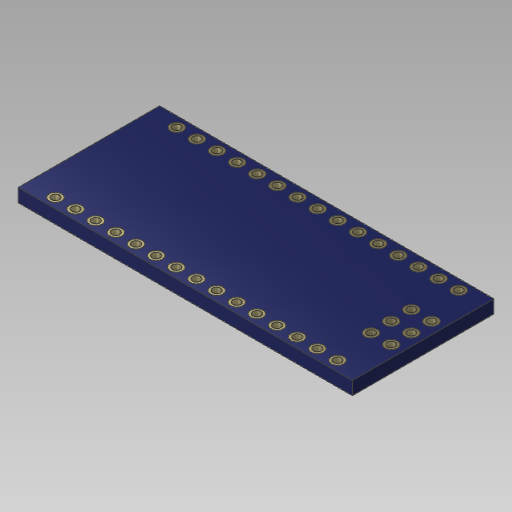
# Autodesk Inventor part: Arduino Nano
Saved by Autodesk Inventor 2020 (Build 240168000, 168)
## iProperties
Created: 2017-10-23
Part Number: Arduino Nano
Material: Generic
Document SubType Name: Modeling
Designer: Alex
Density: 1 g/cm^3
Appearance: Default
Author: Alex
Autodesk Inventor part; units mm, degrees
ref_plane "YZ Plane" through (0, 0, 0) normal (1, 0, 0) x (0, 1, 0)
ref_plane "XZ Plane" through (0, 0, 0) normal (0, 1, 0) x (-1, 0, 0)
ref_plane "XY Plane" through (0, 0, 0) normal (0, 0, 1) x (1, 0, 0)
sketch "Sketch1" plane through (0, 0, 0) normal (0, 1, 0) x (-1, 0, 0)
  line L0 (21.0693, -8.9154) -> (-21.0693, -8.9154)
  line L1 (-21.0693, -8.9154) -> (-21.0693, 8.9154)
  line L2 (-21.0693, 8.9154) -> (21.0693, 8.9154)
  line L3 (21.0693, 8.9154) -> (21.0693, -8.9154)
  line L4 (21.0693, -8.9154) -> (-21.0693, 8.9154) construction
  line L5 (-21.0693, -8.9154) -> (21.0693, 8.9154) construction
  point P0 (0, 0)
  dimension "d0" = 42.1386
  dimension "d1" = 17.8308
  constraints: 12 end point, 2 midpoint, 2 parallel, 1 horizontal, 1 perpendicular
  measures "d0" distance of L1.end L2.end
  measures "d1" distance of L0.end L1.end
extrude "Extrusion1" add sketch "Sketch1" along normal mid plane 1.651
sketch "Sketch2" plane through (0, 0.8255, 0) normal (0, 1, 0) x (1, 0, 0)
  circle A0 centre (-17.6403, 7.6454) radius 0.8001
  line L0 (-21.0693, 8.9154) -> (-21.0693, -8.9154) projected
  line L1 (21.0693, 8.9154) -> (-21.0693, 8.9154) projected
  line L2 (-21.0693, -8.9154) -> (21.0693, -8.9154) projected
  circle A1 centre (-15.1003, 7.6454) radius 0.8001
  circle A2 centre (-12.5603, 7.6454) radius 0.8001
  circle A3 centre (-10.0203, 7.6454) radius 0.8001
  circle A4 centre (-7.4803, 7.6454) radius 0.8001
  circle A5 centre (-4.9403, 7.6454) radius 0.8001
  circle A6 centre (-2.4003, 7.6454) radius 0.8001
  circle A7 centre (0.1397, 7.6454) radius 0.8001
  circle A8 centre (2.6797, 7.6454) radius 0.8001
  circle A9 centre (5.2197, 7.6454) radius 0.8001
  circle A10 centre (7.7597, 7.6454) radius 0.8001
  circle A11 centre (10.2997, 7.6454) radius 0.8001
  circle A12 centre (12.8397, 7.6454) radius 0.8001
  circle A13 centre (15.3797, 7.6454) radius 0.8001
  circle A14 centre (17.9197, 7.6454) radius 0.8001
  line L3 (0, 0) -> (-15.1003, 0) construction
  circle A15 centre (-17.6403, -7.6454) radius 0.8001
  circle A16 centre (-15.1003, -7.6454) radius 0.8001
  circle A17 centre (-12.5603, -7.6454) radius 0.8001
  circle A18 centre (-10.0203, -7.6454) radius 0.8001
  circle A19 centre (-7.4803, -7.6454) radius 0.8001
  circle A20 centre (-4.9403, -7.6454) radius 0.8001
  circle A21 centre (-2.4003, -7.6454) radius 0.8001
  circle A22 centre (0.1397, -7.6454) radius 0.8001
  circle A23 centre (2.6797, -7.6454) radius 0.8001
  circle A24 centre (5.2197, -7.6454) radius 0.8001
  circle A25 centre (7.7597, -7.6454) radius 0.8001
  circle A26 centre (10.2997, -7.6454) radius 0.8001
  circle A27 centre (12.8397, -7.6454) radius 0.8001
  circle A28 centre (15.3797, -7.6454) radius 0.8001
  circle A29 centre (17.9197, -7.6454) radius 0.8001
  circle A30 centre (19.5834, 0) radius 0.8001
  line L4 (21.0693, -8.9154) -> (21.0693, 8.9154) projected
  circle A31 centre (19.5834, -2.54) radius 0.8001
  circle A32 centre (17.0434, 0) radius 0.8001
  circle A33 centre (17.0434, -2.54) radius 0.8001
  circle A34 centre (17.0434, 2.54) radius 0.8001
  circle A35 centre (19.5834, 2.54) radius 0.8001
  dimension "d4" = 1.6002
  dimension "d5" = 3.429
  dimension "d6" = 1.27
  dimension "d7" = 17.8308
  dimension "d10" = 2.54
  dimension "d17" = 1.4859
  dimension "d21" = 2.54
  dimension "d24" = 2.54
  dimension "d29" = 2.54
  constraints: 36 centre point, 15 symmetric about line, 3 horizontal, 2 end point, 2 vertical, 1 equal radius, 1 horizontal alignment, 53 other
  measures "d4" diameter of A0
  measures "d5" distance from line of L0 A0.centre
  measures "d6" distance from line of L1 A0.centre
  measures "d7" distance between parallel lines of L2 L1
  measures "d10" distance of A0.centre A1.centre
  measures "d17" distance from line of L4 A30.centre
  measures "d21" distance of A30.centre A31.centre
  measures "d24" distance of A30.centre A32.centre
  measures "d29" distance of A32.centre A34.centre
extrude "Extrusion2" add sketch "Sketch2" along normal blind 0.0025 contours A0 | A1 | A2 | A3 | A4 | A5 | A6 | A7 | A8 | A9 | A10 | A11 | A12 | A13 | A14 | A15 | A16 | A17 | A18 | A19 | A20 | A21 | A22 | A23 | A24 | A25 | A26 | A27 | A28 | A29 | A30 | A31 | A32 | A33 | A34 | A35
mirror "Mirror1" about plane through (0, 0, 0) normal (0, 1, 0) of "Extrusion2"
sketch "Sketch4" plane through (-17.6403, 0.828, -7.6454) normal (0, 1, 0) x (1, 0, 0)
  circle A0 centre (34.6837, -5.1054) radius 0.8001 projected
  circle A1 centre (34.6837, -7.6454) radius 0.8001 projected
  circle A2 centre (37.2237, -7.6454) radius 0.8001 projected
  circle A3 centre (33.02, -15.2908) radius 0.8001 projected
  circle A4 centre (27.94, -15.2908) radius 0.8001 projected
  circle A5 centre (22.86, -15.2908) radius 0.8001 projected
  circle A6 centre (0, -15.2908) radius 0.8001 projected
  circle A7 centre (2.54, -15.2908) radius 0.8001 projected
  circle A8 centre (10.16, -15.2908) radius 0.8001 projected
  circle A9 centre (15.24, -15.2908) radius 0.8001 projected
  circle A10 centre (35.56, 0) radius 0.8001 projected
  circle A11 centre (30.48, 0) radius 0.8001 projected
  circle A12 centre (25.4, 0) radius 0.8001 projected
  circle A13 centre (20.32, 0) radius 0.8001 projected
  circle A14 centre (15.24, 0) radius 0.8001 projected
  circle A15 centre (10.16, 0) radius 0.8001 projected
  circle A16 centre (5.08, 0) radius 0.8001 projected
  circle A17 centre (0, 0) radius 0.8001 projected
  circle A18 centre (2.54, 0) radius 0.8001 projected
  circle A19 centre (7.62, 0) radius 0.8001 projected
  circle A20 centre (12.7, 0) radius 0.8001 projected
  circle A21 centre (17.78, 0) radius 0.8001 projected
  circle A22 centre (22.86, 0) radius 0.8001 projected
  circle A23 centre (27.94, 0) radius 0.8001 projected
  circle A24 centre (33.02, 0) radius 0.8001 projected
  circle A25 centre (17.78, -15.2908) radius 0.8001 projected
  circle A26 centre (12.7, -15.2908) radius 0.8001 projected
  circle A27 centre (7.62, -15.2908) radius 0.8001 projected
  circle A28 centre (5.08, -15.2908) radius 0.8001 projected
  circle A29 centre (20.32, -15.2908) radius 0.8001 projected
  circle A30 centre (25.4, -15.2908) radius 0.8001 projected
  circle A31 centre (30.48, -15.2908) radius 0.8001 projected
  circle A32 centre (35.56, -15.2908) radius 0.8001 projected
  circle A33 centre (37.2237, -10.1854) radius 0.8001 projected
  circle A34 centre (34.6837, -10.1854) radius 0.8001 projected
  circle A35 centre (37.2237, -5.1054) radius 0.8001 projected
  line L0 (38.7096, 1.27) -> (-3.429, 1.27) projected
  line L1 (-3.429, 1.27) -> (-3.429, -16.5608) projected
  line L2 (-3.429, -16.5608) -> (38.7096, -16.5608) projected
  line L3 (38.7096, -16.5608) -> (38.7096, 1.27) projected
  point P0 (17.6403, -7.6454)
hole "Hole1" at (0.1397, 0.828, 7.6454) at (2.6797, 0.828, 7.6454) at (-7.4803, 0.828, -7.6454) at (-2.4003, 0.828, -7.6454) at (-4.9403, 0.828, -7.6454) at (0.1397, 0.828, -7.6454) at (5.2197, 0.828, 7.6454) at (2.6797, 0.828, -7.6454) at (7.7597, 0.828, 7.6454) at (5.2197, 0.828, -7.6454) at (10.2997, 0.828, 7.6454) at (15.3797, 0.828, 7.6454) at (17.0434, 0.828, -2.54) at (-2.4003, 0.828, 7.6454) at (17.0434, 0.828, 0) at (19.5834, 0.828, 0) at (7.7597, 0.828, -7.6454) at (12.8397, 0.828, -7.6454) at (17.9197, 0.828, -7.6454) at (-17.6403, 0.828, 7.6454) at (-15.1003, 0.828, 7.6454) at (-10.0203, 0.828, 7.6454) at (-12.5603, 0.828, 7.6454) at (-10.0203, 0.828, -7.6454) at (-12.5603, 0.828, -7.6454) at (-15.1003, 0.828, -7.6454) at (-17.6403, 0.828, -7.6454) at (-7.4803, 0.828, 7.6454) at (-4.9403, 0.828, 7.6454) at (10.2997, 0.828, -7.6454) at (12.8397, 0.828, 7.6454) at (15.3797, 0.828, -7.6454) at (17.9197, 0.828, 7.6454) at (19.5834, 0.828, 2.54) at (19.5834, 0.828, -2.54) at (17.0434, 0.828, 2.54) direction (0, -1, 0) diameter 1.016 end through all
sketch "Sketch5" plane through (0, -0.8255, 0) normal (0, -1, 0) x (1, 0, 0)
  line L0 (-1.6129, 0) -> (-6.2611, 4.6482)
  line L1 (-6.2611, 4.6482) -> (-10.9093, 0)
  line L2 (-10.9093, 0) -> (-6.2611, -4.6482)
  line L3 (-6.2611, -4.6482) -> (-1.6129, 0)
  line L4 (-21.0693, 8.9154) -> (-21.0693, -8.9154) projected
  point P0 (0, 0)
  dimension "d45" = 9.2964
  dimension "d46" = 10.16
  constraints: 8 end point, 2 horizontal alignment, 2 parallel, 1 perpendicular, 1 vertical alignment
  measures "d45" distance of L1.end L0.start
  measures "d46" distance from line of L4 L1.end
extrude "Extrusion3" add sketch "Sketch5" along normal blind 1.143
sketch "Sketch6" plane through (-6.2611, -1.9685, -4.6482) normal (-0.7071, 0, -0.7071) x (-0.7071, 0, 0.7071)
  line L0 (0.508, 0.381) -> (0.889, 0.381)
  line L1 (0.889, 0.381) -> (0.889, 0.254)
  line L2 (0.889, 0.254) -> (0.508, 0.254)
  line L3 (0.508, 0.254) -> (0.508, 0.381)
  line L4 (6.5735, 0) -> (0, 0) projected
  line L5 (0, 1.143) -> (0, 0) projected
  line L6 (1.2475, 0.381) -> (1.6285, 0.381)
  line L7 (1.6285, 0.381) -> (1.6285, 0.254)
  line L8 (1.6285, 0.254) -> (1.2475, 0.254)
  line L9 (1.2475, 0.254) -> (1.2475, 0.381)
  line L10 (1.987, 0.381) -> (2.368, 0.381)
  line L11 (2.368, 0.381) -> (2.368, 0.254)
  line L12 (2.368, 0.254) -> (1.987, 0.254)
  line L13 (1.987, 0.254) -> (1.987, 0.381)
  line L14 (2.7265, 0.381) -> (3.1075, 0.381)
  line L15 (3.1075, 0.381) -> (3.1075, 0.254)
  line L16 (3.1075, 0.254) -> (2.7265, 0.254)
  line L17 (2.7265, 0.254) -> (2.7265, 0.381)
  line L18 (3.466, 0.381) -> (3.847, 0.381)
  line L19 (3.847, 0.381) -> (3.847, 0.254)
  line L20 (3.847, 0.254) -> (3.466, 0.254)
  line L21 (3.466, 0.254) -> (3.466, 0.381)
  line L22 (4.2055, 0.381) -> (4.5865, 0.381)
  line L23 (4.5865, 0.381) -> (4.5865, 0.254)
  line L24 (4.5865, 0.254) -> (4.2055, 0.254)
  line L25 (4.2055, 0.254) -> (4.2055, 0.381)
  line L26 (4.945, 0.381) -> (5.326, 0.381)
  line L27 (5.326, 0.381) -> (5.326, 0.254)
  line L28 (5.326, 0.254) -> (4.945, 0.254)
  line L29 (4.945, 0.254) -> (4.945, 0.381)
  line L30 (5.6845, 0.381) -> (6.0655, 0.381)
  line L31 (6.0655, 0.381) -> (6.0655, 0.254)
  line L32 (6.0655, 0.254) -> (5.6845, 0.254)
  line L33 (5.6845, 0.254) -> (5.6845, 0.381)
  point P0 (-1.1405, 1.9685)
  dimension "d49" = 0.381
  dimension "d50" = 0.127
  dimension "d51" = 0.254
  dimension "d52" = 0.508
  dimension "d53" = 6.5736
  dimension "d56" = 0.7395
  constraints: 64 end point, 2 horizontal, 2 parallel, 1 perpendicular, 56 other
  measures "d49" distance of L1.end L2.end
  measures "d50" distance of L2.end L0.start
  measures "d51" distance between parallel lines of L4 L2
  measures "d52" distance between parallel lines of L5 L3
  measures "d53" distance of L4.start L4.end
  measures "d56" distance of L0.start L6.start
sketch "Sketch7" plane through (-1.6129, -1.9685, 0) normal (0.7071, 0, -0.7071) x (-0.7071, 0, -0.7071)
  line L0 (6.5735, 1.143) -> (6.5735, 0) projected
  line L1 (6.5735, 0.3175) -> (6.9545, 0.3175)
  arc A0 (6.9545, 0.3175) -> (7.2584, 0.6466) centre (6.9545, 0.6223) ccw
  arc A1 (7.7165, 1.143) -> (7.2584, 0.6466) centre (7.7165, 0.6834) ccw
  line L2 (20.0619, 1.143) -> (-9.7346, 1.143) projected
  line L3 (6.5735, 0.381) -> (6.5735, 0.254) projected
  point P0 (-1.1405, 1.9685)
  dimension "d61" = 0.381
  dimension "d62" = 0.3048
  dimension "d63" = 1.143
  constraints: 4 point on circle, 3 tangent, 2 centre point, 2 end point, 1 midpoint, 1 perpendicular, 1 point on line
  measures "d61" distance of L1.start L1.end
  measures "d62" radius of A0
  measures "d63" distance from line of L0 A1.centre
sweep "Sweep1" add profiles "Sketch6" path "Sketch7" path curves A1 A0 L1
sketch "Sketch8" plane through (0, -1.9685, 0) normal (0, -1, 0) x (1, 0, 0)
  line L0 (-1.6129, 0) -> (-6.2611, 4.6482) construction
  line L1 (-6.2611, 4.6482) -> (-10.9093, 0) construction
  line L2 (-10.9093, 0) -> (-6.2611, -4.6482) construction
  line L3 (-6.2611, -4.6482) -> (-1.6129, 0) construction
  line L4 (-10.9093, 0) -> (-6.2611, -4.6482) construction
  line L5 (-10.9093, 0) -> (-1.6129, 0) construction
  point P0 (0, 0)
  point P1 (-6.2611, 0)
  constraints: 2 end point, 1 horizontal, 1 midpoint
pattern_circular "Circular Pattern1" count 4 over 360 about axis through (-6.2611, -1.9685, 0) along (0, -1, 0) of "Sweep1"
sketch "Sketch9" plane through (0, -0.8255, 0) normal (0, -1, 0) x (1, 0, 0)
  line L0 (-1.4333, -1.4368) -> (-1.1639, -1.1674) construction
  line L1 (-1.6099, -1.2602) -> (-1.3405, -0.9908) construction
  line L2 (-1.6099, -1.2602) -> (-1.802, -1.0681) construction
  line L3 (-1.5326, -0.7987) -> (-1.802, -1.0681) construction
  line L4 (-1.3405, -0.9908) -> (-1.5326, -0.7987) construction
  line L5 (-1.0646, -1.8056) -> (-1.802, -1.0681)
  line L6 (-1.802, -1.0681) -> (-1.5326, -0.7987)
  line L7 (-1.5326, -0.7987) -> (-0.7952, -1.5362)
  line L8 (-0.7952, -1.5362) -> (-1.0646, -1.8056)
  line L9 (-0.6694, -1.5901) -> (-1.5865, -0.673)
  line L10 (-1.5865, -0.673) -> (-1.9278, -1.0142)
  line L11 (-1.9278, -1.0142) -> (-1.0107, -1.9313)
  line L12 (-1.0107, -1.9313) -> (-0.6694, -1.5901)
  line L13 (-1.0107, -1.9313) -> (-1.5865, -0.673) construction
  line L14 (-1.9278, -1.0142) -> (-0.6694, -1.5901) construction
  line L15 (-1.6868, -1.6903) -> (-1.9669, -1.4102) projected
  line L16 (-1.9562, -1.9598) -> (-2.2363, -1.6796) projected
  point P0 (0, 0)
  point P1 (-1.2986, -1.3021)
  point P2 (-1.966, -1.4111)
  point P3 (-2.2354, -1.6805)
  dimension "d69" = 0.127
  dimension "d70" = 0.0508
  dimension "d73" = 0.3585
  dimension "d74" = 0.381
  constraints: 20 end point, 5 parallel, 4 midpoint, 2 perpendicular
  measures "d69" distance between parallel lines of L8 L12
  measures "d70" distance between parallel lines of L11 L5
  measures "d73" distance between parallel lines of L5 L15
  measures "d74" distance between parallel lines of L16 L15
extrude "Extrusion4" add sketch "Sketch9" along normal blind 0.0025 contours L5 L6 L7 L8 | L12 L11 L10 L9
pattern_linear "Rectangular Pattern1" count 8 spacing 0.7395 along (-0.7071, 0, -0.7071) of "Extrusion4"
pattern_circular "Circular Pattern2" count 4 over 360 about axis through (-6.2611, -1.9685, 0) along (0, -1, 0) of "Extrusion4", "Rectangular Pattern1"
sketch "Sketch10" plane through (0, -0.8255, 0) normal (0, -1, 0) x (1, 0, 0)
  line L0 (8.0193, 3.3604) -> (8.0193, 4.1204) projected
  line L1 (9.5693, 4.1204) -> (9.5693, 3.3604) projected
  line L2 (9.2693, 4.1679) -> (8.3193, 4.1679) projected
  line L3 (9.2693, 1.6679) -> (8.3193, 1.6679) projected
  line L4 (10.8393, 4.1654) -> (10.8393, 3.2654) projected
  line L5 (12.5393, 4.1654) -> (12.5393, 3.2654) projected
  line L6 (12.1485, 4.1604) -> (11.2301, 4.1604) projected
  line L7 (12.1485, 1.6604) -> (11.2301, 1.6604) projected
  line L8 (8.3241, 4.2949) -> (7.8161, 4.2949)
  line L9 (7.8161, 4.2949) -> (7.8161, 3.1859)
  line L10 (7.8161, 3.1859) -> (8.3241, 3.1859)
  line L11 (8.3241, 3.1859) -> (8.3241, 4.2949)
  line L12 (8.3241, 4.2949) -> (7.8161, 3.1859) construction
  line L13 (7.8161, 4.2949) -> (8.3241, 3.1859) construction
  line L14 (9.7725, 4.2949) -> (9.2645, 4.2949)
  line L15 (9.2645, 4.2949) -> (9.2645, 3.1859)
  line L16 (9.2645, 3.1859) -> (9.7725, 3.1859)
  line L17 (9.7725, 3.1859) -> (9.7725, 4.2949)
  line L18 (9.7725, 4.2949) -> (9.2645, 3.1859) construction
  line L19 (9.2645, 4.2949) -> (9.7725, 3.1859) construction
  line L20 (8.7943, 4.1679) -> (8.7943, 2.8923) construction
  line L21 (11.6893, 4.1604) -> (11.6893, 3.1364) construction
  line L22 (10.6361, 4.2699) -> (11.1441, 4.2699)
  line L23 (11.1441, 4.2699) -> (11.1441, 3.1609)
  line L24 (11.1441, 3.1609) -> (10.6361, 3.1609)
  line L25 (10.6361, 3.1609) -> (10.6361, 4.2699)
  line L26 (10.6361, 4.2699) -> (11.1441, 3.1609) construction
  line L27 (11.1441, 4.2699) -> (10.6361, 3.1609) construction
  line L28 (12.5393, 4.1654) -> (12.5393, 3.2654)
  line L29 (12.7425, 4.2699) -> (12.2345, 4.2699)
  line L30 (12.2345, 4.2699) -> (12.2345, 3.1609)
  line L31 (12.2345, 3.1609) -> (12.7425, 3.1609)
  line L32 (12.7425, 3.1609) -> (12.7425, 4.2699)
  line L33 (12.7425, 4.2699) -> (12.2345, 3.1609) construction
  line L34 (12.2345, 4.2699) -> (12.7425, 3.1609) construction
  line L35 (9.2645, 0.6859) -> (9.7725, 0.6859)
  line L36 (10.6361, 0.6609) -> (10.6361, 1.7699)
  line L37 (10.6361, 1.7699) -> (11.1441, 1.7699)
  line L38 (11.1441, 1.7699) -> (11.1441, 0.6609)
  line L39 (10.6361, 1.7699) -> (11.1441, 0.6609) construction
  line L40 (11.1441, 1.7699) -> (10.6361, 0.6609) construction
  line L41 (11.1441, 0.6609) -> (10.6361, 0.6609)
  line L42 (12.2345, 1.7699) -> (12.2345, 0.6609)
  line L43 (12.2345, 0.6609) -> (12.7425, 0.6609)
  line L44 (12.7425, 0.6609) -> (12.7425, 1.7699)
  line L45 (12.7425, 1.7699) -> (12.2345, 0.6609) construction
  line L46 (12.2345, 1.7699) -> (12.7425, 0.6609) construction
  line L47 (12.7425, 1.7699) -> (12.2345, 1.7699)
  line L48 (9.7725, 0.6859) -> (9.7725, 1.7949)
  line L49 (9.7725, 1.7949) -> (9.2645, 0.6859) construction
  line L50 (9.2645, 1.7949) -> (9.7725, 0.6859) construction
  line L51 (9.7725, 1.7949) -> (9.2645, 1.7949)
  line L52 (7.8161, 0.6859) -> (8.3241, 0.6859)
  line L53 (9.2645, 1.7949) -> (9.2645, 0.6859)
  line L54 (8.3241, 0.6859) -> (8.3241, 1.7949)
  line L55 (8.3241, 1.7949) -> (7.8161, 1.7949)
  line L56 (8.3241, 1.7949) -> (7.8161, 0.6859) construction
  line L57 (7.8161, 1.7949) -> (8.3241, 0.6859) construction
  line L58 (7.8161, 1.7949) -> (7.8161, 0.6859)
  line L59 (9.2645, -1.8141) -> (9.7725, -1.8141)
  line L60 (10.6361, -1.8391) -> (10.6361, -0.7301)
  line L61 (10.6361, -0.7301) -> (11.1441, -0.7301)
  line L62 (11.1441, -0.7301) -> (11.1441, -1.8391)
  line L63 (10.6361, -0.7301) -> (11.1441, -1.8391) construction
  line L64 (11.1441, -0.7301) -> (10.6361, -1.8391) construction
  line L65 (11.1441, -1.8391) -> (10.6361, -1.8391)
  line L66 (12.2345, -0.7301) -> (12.2345, -1.8391)
  line L67 (12.2345, -1.8391) -> (12.7425, -1.8391)
  line L68 (12.7425, -1.8391) -> (12.7425, -0.7301)
  line L69 (12.7425, -0.7301) -> (12.2345, -1.8391) construction
  line L70 (12.2345, -0.7301) -> (12.7425, -1.8391) construction
  line L71 (12.7425, -0.7301) -> (12.2345, -0.7301)
  line L72 (9.7725, -1.8141) -> (9.7725, -0.7051)
  line L73 (9.7725, -0.7051) -> (9.2645, -1.8141) construction
  line L74 (9.2645, -0.7051) -> (9.7725, -1.8141) construction
  line L75 (9.7725, -0.7051) -> (9.2645, -0.7051)
  line L76 (7.8161, -1.8141) -> (8.3241, -1.8141)
  line L77 (9.2645, -0.7051) -> (9.2645, -1.8141)
  line L78 (8.3241, -1.8141) -> (8.3241, -0.7051)
  line L79 (8.3241, -0.7051) -> (7.8161, -0.7051)
  line L80 (8.3241, -0.7051) -> (7.8161, -1.8141) construction
  line L81 (7.8161, -0.7051) -> (8.3241, -1.8141) construction
  line L82 (7.8161, -0.7051) -> (7.8161, -1.8141)
  line L83 (9.2645, -4.3141) -> (9.7725, -4.3141)
  line L84 (10.6361, -4.3391) -> (10.6361, -3.2301)
  line L85 (10.6361, -3.2301) -> (11.1441, -3.2301)
  line L86 (11.1441, -3.2301) -> (11.1441, -4.3391)
  line L87 (10.6361, -3.2301) -> (11.1441, -4.3391) construction
  line L88 (11.1441, -3.2301) -> (10.6361, -4.3391) construction
  line L89 (11.1441, -4.3391) -> (10.6361, -4.3391)
  line L90 (12.2345, -3.2301) -> (12.2345, -4.3391)
  line L91 (12.2345, -4.3391) -> (12.7425, -4.3391)
  line L92 (12.7425, -4.3391) -> (12.7425, -3.2301)
  line L93 (12.7425, -3.2301) -> (12.2345, -4.3391) construction
  line L94 (12.2345, -3.2301) -> (12.7425, -4.3391) construction
  line L95 (12.7425, -3.2301) -> (12.2345, -3.2301)
  line L96 (9.7725, -4.3141) -> (9.7725, -3.2051)
  line L97 (9.7725, -3.2051) -> (9.2645, -4.3141) construction
  line L98 (9.2645, -3.2051) -> (9.7725, -4.3141) construction
  line L99 (9.7725, -3.2051) -> (9.2645, -3.2051)
  line L100 (7.8161, -4.3141) -> (8.3241, -4.3141)
  line L101 (9.2645, -3.2051) -> (9.2645, -4.3141)
  line L102 (8.3241, -4.3141) -> (8.3241, -3.2051)
  line L103 (8.3241, -3.2051) -> (7.8161, -3.2051)
  line L104 (8.3241, -3.2051) -> (7.8161, -4.3141) construction
  line L105 (7.8161, -3.2051) -> (8.3241, -4.3141) construction
  line L106 (7.8161, -3.2051) -> (7.8161, -4.3141)
  line L107 (3.7274, 4.064) -> (4.2354, 4.064) projected
  line L108 (5.8293, 3.048) -> (2.1336, 3.048) projected
  line L109 (4.4894, 4.318) -> (3.4734, 4.318)
  line L110 (3.4734, 4.318) -> (3.4734, 3.048)
  line L111 (3.4734, 3.048) -> (4.4894, 3.048)
  line L112 (4.4894, 3.048) -> (4.4894, 4.318)
  line L113 (4.4894, 4.318) -> (3.4734, 3.048) construction
  line L114 (3.4734, 4.318) -> (4.4894, 3.048) construction
  line L115 (2.1336, 3.048) -> (2.1336, -3.048) projected
  line L116 (2.1336, 0) -> (6.3479, 0)
  line L117 (3.7274, -4.064) -> (4.2354, -4.064)
  line L118 (4.4894, -4.318) -> (3.4734, -4.318)
  line L119 (3.4734, -4.318) -> (3.4734, -3.048)
  line L120 (3.4734, -3.048) -> (4.4894, -3.048)
  line L121 (4.4894, -3.048) -> (4.4894, -4.318)
  line L122 (4.4894, -4.318) -> (3.4734, -3.048) construction
  line L123 (3.4734, -4.318) -> (4.4894, -3.048) construction
  point P0 (0, 0)
  point P1 (8.0701, 3.7404)
  point P2 (8.0701, 3.7404)
  point P3 (8.0193, 3.7404)
  point P4 (9.5185, 3.7404)
  point P5 (10.8901, 3.7154)
  point P6 (10.8901, 3.7154)
  point P7 (10.8393, 3.7154)
  point P8 (12.4885, 3.7154)
  point P9 (12.4885, 3.7154)
  point P10 (12.5393, 3.7154)
  point P11 (8.0701, 1.2404)
  point P12 (10.8901, 1.2154)
  point P13 (12.4885, 1.2154)
  point P14 (8.0701, 1.2404)
  point P15 (9.2693, 1.6679)
  point P16 (8.3193, 1.6679)
  point P17 (8.0701, -1.2596)
  point P18 (10.8901, -1.2846)
  point P19 (12.4885, -1.2846)
  point P20 (8.0701, -1.2596)
  point P21 (9.2693, -0.8321)
  point P22 (8.3193, -0.8321)
  point P23 (8.0701, -3.7596)
  point P24 (10.8901, -3.7846)
  point P25 (12.4885, -3.7846)
  point P26 (8.0701, -3.7596)
  point P27 (9.2693, -3.3321)
  point P28 (8.3193, -3.3321)
  point P29 (3.9814, 3.683)
  point P30 (3.9814, 3.683)
  point P31 (3.9814, 4.064)
  point P32 (3.9814, -3.683)
  point P33 (3.9814, -3.683)
  point P34 (3.9814, -4.064)
  dimension "d81" = 0.127
  dimension "d82" = 0.508
  dimension "d83" = 0.2032
  dimension "d84" = 0.2032
  dimension "d85" = 2.5
  dimension "d88" = 2.5
  dimension "d93" = 0.254
  dimension "d94" = 0.254
  constraints: 226 end point, 27 midpoint, 16 symmetric about line, 8 parallel, 5 horizontal, 4 equal length, 4 perpendicular, 3 horizontal alignment, 3 vertical, 1 collinear, 1 point on line, 1 vertical alignment, 138 other
  measures "d81" distance between parallel lines of L8 L2
  measures "d82" distance of L8.start L8.end
  measures "d83" distance between parallel lines of L0 L9
  measures "d84" distance between parallel lines of L25 L4
  measures "d85" distance between parallel lines of L3 L2
  measures "d88" distance of L15.end L35.start
  measures "d93" distance from line of L107.start L110
  measures "d94" distance between parallel lines of L109 L107
extrude "Extrusion5" add sketch "Sketch10" along normal blind 0.0025
equation "\"d56\" = -0.142857 * d49 + 0.142857 * d53 - 0.285714 * d52"
equation "\"d77\" = d74 + d73"
equation "\"d83\" = 0.4 * d82"
equation "\"d84\" = d83"
equation "\"d88\" = d85"
body "Solid1"
